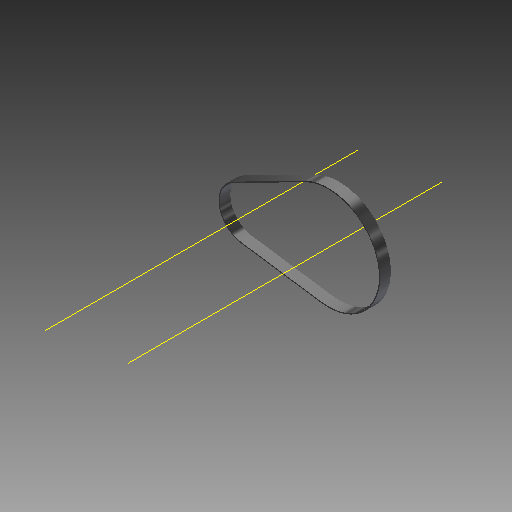
# Autodesk Inventor part: Synchronous Belt
Saved by Autodesk Inventor 2019.4 (Build 234330000, 330)
## iProperties
Created: 2020-01-18
Part Number: Synchronous Belt
Material: Rubber
Document SubType Name: Modeling
Designer: admin
Density: 0.93 g/cm^3
Appearance: Rubber - Black - Version 1.1
Mass: 3.627 g
Surface Area: 85.8 cm^2
Volume: 3.9 cm^3
CustomPartVersion: 1
Author: admin
Autodesk Inventor part; units mm, degrees
sketch "Sketch Path" plane through (0, 0, 0) normal (0, 0, 1) x (1, 0, 0)
  arc A0 (-169.5723, -46.5624) -> (-162.1462, -91.4584) centre (-158.7288, -67.831) ccw
  arc A1 (-87.7627, -102.2169) -> (-102.6149, -12.4251) centre (-80.9279, -54.9621) ccw
  line L0 (-87.7627, -102.2169) -> (-162.1462, -91.4584)
  line L1 (-169.5723, -46.5624) -> (-102.6149, -12.4251)
  constraints: 4 end point, 4 point on circle, 2 centre point
ref_plane "Cross Section Plane" through (-162.1462, -91.4584, 0) normal (0.9897, -0.1431, 0) x (0, 0, 1)
ref_plane "Work Plane2" through (-158.7288, -67.831, 0) normal (-1, 0, 0) x (0, 0, 1)
ref_plane "Work Plane3" through (-80.9279, -54.9621, 0) normal (-0.9011, -0.4336, 0) x (0, 0, 1)
sketch "Cross Section" plane through (-162.1462, -91.4584, 0) normal (0.9897, -0.1431, 0) x (0, 0, 1)
  line L0 (-5, 0.5) -> (5, 0.5)
  line L1 (5, 0.5) -> (5, -0.5)
  line L2 (5, -0.5) -> (-5, -0.5)
  line L3 (-5, -0.5) -> (-5, 0.5)
  line L4 (-5, 0) -> (5, 0) construction
  point P0 (0, 0)
  point P1 (0, 0)
  dimension "d0" = 10
  dimension "d4" = 0.5
  dimension "d5" = 0.5
  constraints: 10 end point, 3 midpoint, 2 parallel, 1 coincident, 1 horizontal, 1 perpendicular, 1 other
  measures "d0" distance between parallel lines of L1 L3
  measures "d4" distance between parallel lines of L2 L4
  measures "d5" distance between parallel lines of L4 L0
sweep "Belt" add profiles "Cross Section" path "Sketch Path"
equation "\"d0\" = da_B"
equation "\"d4\" = da_a"
equation "\"d5\" = da_a2"
equation "\"da_B\" = 10"
equation "\"da_pb\" = 5"
equation "\"da_L\" = 390.0001"
equation "\"da_a\" = 0.5"
equation "\"da_S\" = 2.65"
equation "\"da_Beta\" = 20deg"
equation "\"da_Ht\" = 1.2"
equation "\"da_H\" = 2.2"
equation "\"da_a2\" = 0.5"
body "Solid1"
